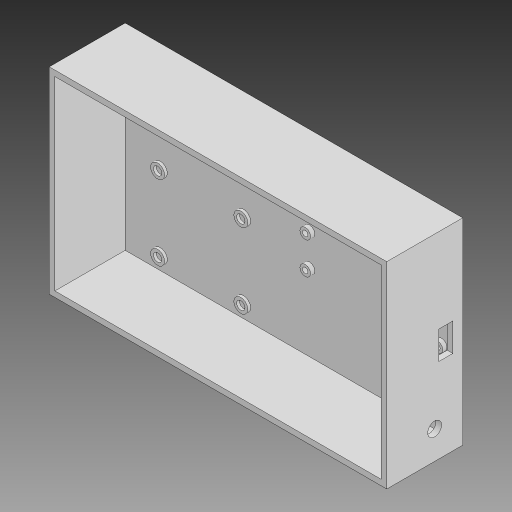
# Autodesk Inventor part: box
Saved by Autodesk Inventor 2023 (Build 270158000, 158)
## iProperties
Created: 2024-01-29
Part Number: box
Material: Všeobecné
Document SubType Name: Modeling
Designer: matej
Mass: 35.3602 g
Surface Area: 363.22 cm^2
Volume: 35.3602 cm^3
Density: 1 g/cm^3
Appearance: Výchozí
Author: matej
Autodesk Inventor part; units mm, degrees
ref_plane "YZ Plane" through (0, 0, 0) normal (1, 0, 0) x (0, 1, 0)
ref_plane "XZ Plane" through (0, 0, 0) normal (0, 1, 0) x (-1, 0, 0)
ref_plane "XY Plane" through (0, 0, 0) normal (0, 0, 1) x (1, 0, 0)
sketch "Náčrt1" plane through (0, 0, 0) normal (0, 0, 1) x (1, 0, 0)
  line L0 (-60, -35) -> (60, -35)
  line L1 (60, -35) -> (60, 35)
  line L2 (60, 35) -> (-60, 35)
  line L3 (-60, 35) -> (-60, -35)
  line L4 (-60, -35) -> (60, 35) construction
  line L5 (60, -35) -> (-60, 35) construction
  point P0 (0, 0)
  dimension "d0" = 120
  dimension "d1" = 70
  constraints: 12 end point, 2 midpoint, 2 parallel, 1 horizontal, 1 perpendicular
  measures "d0" distance of L2.end L1.end
  measures "d1" distance of L1.end L0.end
extrude "Vysunutí1" add sketch "Náčrt1" along normal blind 2
sketch "Náčrt2" plane through (0, 0, 2) normal (0, 0, 1) x (1, 0, 0)
  line L0 (60, -35) -> (60, 35) projected
  line L1 (-60, -35) -> (60, -35)
  line L2 (60, -35) -> (60, 35)
  line L3 (60, 35) -> (-60, 35)
  line L4 (-60, 35) -> (-60, -35)
  line L5 (-60, -35) -> (60, 35) construction
  line L6 (60, -35) -> (-60, 35) construction
  line L7 (-58, -33) -> (58, -33)
  line L8 (58, -33) -> (58, 33)
  line L9 (58, 33) -> (-58, 33)
  line L10 (-58, 33) -> (-58, -33)
  line L11 (-58, -33) -> (58, 33) construction
  line L12 (58, -33) -> (-58, 33) construction
  point P0 (0, 0)
  point P1 (60, -35)
  dimension "d4" = 116
  dimension "d5" = 66
  constraints: 24 end point, 4 midpoint, 4 parallel, 2 horizontal, 2 perpendicular
  measures "d4" distance of L9.end L8.end
  measures "d5" distance of L8.end L7.end
extrude "Vysunutí2" add sketch "Náčrt2" along normal blind 25
sketch "Náčrt3" plane through (60, -35, 0) normal (1, 0, 0) x (0, 0, -1)
  line L0 (-8.5, 30) -> (-3.5, 30)
  line L1 (-3.5, 30) -> (-3.5, 40)
  line L2 (-3.5, 40) -> (-8.5, 40)
  line L3 (-8.5, 40) -> (-8.5, 30)
  line L4 (-8.5, 30) -> (-3.5, 40) construction
  line L5 (-3.5, 30) -> (-8.5, 40) construction
  line L6 (0, 0) -> (0, 70) projected
  point P0 (0, 35)
  point P1 (-6, 35)
  point P2 (0, 35)
  dimension "d8" = 3.5
  dimension "d9" = 5
  dimension "d10" = 10
  constraints: 12 end point, 3 midpoint, 2 parallel, 1 horizontal, 1 horizontal alignment, 1 perpendicular
  measures "d8" distance between parallel lines of L1 L6
  measures "d9" distance of L0.start L0.end
  measures "d10" distance of L2.end L0.start
extrude "micro usb hole" cut sketch "Náčrt3" against normal blind 5
sketch "Náčrt4" plane through (0, 0, 2) normal (0, 0, 1) x (1, 0, 0)
  circle A0 centre (54.5, 5.7) radius 1.9
  circle A1 centre (54.5, -5.7) radius 1.9
  circle A2 centre (7.5, 5.7) radius 1.9
  circle A3 centre (7.5, -5.7) radius 1.9
  line L0 (5.5, 10.5) -> (56.5, 10.5)
  line L1 (56.5, 10.5) -> (56.5, -10.5)
  line L2 (56.5, -10.5) -> (5.5, -10.5)
  line L3 (5.5, -10.5) -> (5.5, 10.5)
  line L4 (60, -35) -> (60, 35) projected
  line L5 (58, 33) -> (58, -33) projected
  circle A4 centre (54.5, 5.7) radius 1
  circle A5 centre (7.5, 5.7) radius 1
  circle A6 centre (7.5, -5.7) radius 1
  circle A7 centre (54.5, -5.7) radius 1
  point P0 (0, 0)
  point P1 (56.5, 0)
  point P2 (60, 0)
  dimension "d13" = 3.8
  dimension "d14" = 3.8
  dimension "d15" = 11.4
  dimension "d16" = 3.8
  dimension "d18" = 3.8
  dimension "d19" = 51
  dimension "d20" = 2
  dimension "d21" = 2
  dimension "d22" = 21
  dimension "d23" = 4.8
  dimension "d24" = 1.5
  dimension "d25" = 2
  dimension "d26" = 2
  dimension "d27" = 2
  dimension "d28" = 2
  constraints: 8 centre point, 8 end point, 4 coincident, 3 horizontal alignment, 2 midpoint, 2 parallel, 2 vertical alignment, 1 horizontal, 1 perpendicular
  measures "d13" diameter of A0
  measures "d14" diameter of A1
  measures "d15" distance of A1.centre A0.centre
  measures "d16" diameter of A2
  measures "d18" diameter of A3
  measures "d19" distance of L0.start L0.end
  measures "d20" distance from line of L1 A0.centre
  measures "d21" distance from line of L3 A2.centre
  measures "d22" distance of L2.end L0.start
  measures "d23" distance from line of L0 A0.centre
  measures "d24" distance between parallel lines of L5 L1
  measures "d25" diameter of A4
  measures "d26" diameter of A5
  measures "d27" diameter of A6
  measures "d28" diameter of A7
extrude "rpi holder" add sketch "Náčrt4" along normal blind 1.5 contours A0 | A1 | A2 | A3
sketch "Náčrt6" plane through (60, -35, 0) normal (1, 0, 0) x (0, 0, -1)
  circle A0 centre (-10, 10) radius 2.5
  line L0 (0, 70) -> (-27, 70) projected
  line L1 (0, 0) -> (0, 70) projected
  line L2 (0, 0) -> (-27, 0) projected
  point P0 (0, 35)
  dimension "d36" = 5
  dimension "d38" = 10
  dimension "d59" = 10
  constraints: 1 centre point
  measures "d36" diameter of A0
  measures "d38" distance from line of L1 A0.centre
  measures "d59" distance from line of L2 A0.centre
extrude "rgb led hole" cut sketch "Náčrt6" against normal blind 10
sketch "Náčrt7" plane through (0, 0, 2) normal (0, 0, 1) x (1, 0, 0)
  line L0 (-48, 0.8) -> (-13.4, 0.8)
  line L1 (-13.4, 0.8) -> (-13.4, -31)
  line L2 (-13.4, -31) -> (-48, -31)
  line L3 (-48, -31) -> (-48, 0.8)
  circle A0 centre (-15.9, -1.8) radius 1.5
  circle A1 centre (-45.5, -1.8) radius 2.5
  circle A2 centre (-45.5, -28.4) radius 1.5
  circle A3 centre (-15.9, -28.4) radius 1.5
  circle A4 centre (-45.5, -1.8) radius 1.5
  circle A5 centre (-15.9, -1.8) radius 2.5
  circle A6 centre (-15.9, -28.4) radius 2.5
  circle A7 centre (-45.5, -28.4) radius 2.5
  line L4 (-58, -33) -> (-58, 33) projected
  line L5 (58, -33) -> (-58, -33) projected
  point P0 (0, 0)
  point P1 (-48, -1.8)
  point P2 (-48, -28.4)
  point P3 (-13.4, -28.4)
  point P4 (-13.4, -1.8)
  dimension "d41" = 34.6
  dimension "d42" = 31.8
  dimension "d43" = 3
  dimension "d44" = 5
  dimension "d45" = 29.6
  dimension "d46" = 2.5
  dimension "d47" = 2.6
  dimension "d48" = 3
  dimension "d49" = 3
  dimension "d50" = 26.6
  dimension "d51" = 3
  dimension "d52" = 5
  dimension "d53" = 5
  dimension "d54" = 5
  dimension "d55" = 10
  dimension "d56" = 2
  constraints: 8 centre point, 8 end point, 4 coincident, 2 horizontal alignment, 2 parallel, 2 vertical alignment, 1 horizontal, 1 perpendicular
  measures "d41" distance of L1.end L2.end
  measures "d42" distance of L0.end L1.end
  measures "d43" diameter of A0
  measures "d44" diameter of A1
  measures "d45" distance of A1.centre A0.centre
  measures "d46" distance from line of L1 A0.centre
  measures "d47" distance from line of L0 A0.centre
  measures "d48" diameter of A2
  measures "d49" diameter of A3
  measures "d50" distance of A0.centre A3.centre
  measures "d51" diameter of A4
  measures "d52" diameter of A5
  measures "d53" diameter of A6
  measures "d54" diameter of A7
  measures "d55" distance between parallel lines of L4 L3
  measures "d56" distance between parallel lines of L5 L2
extrude "ULN2003 holder" add sketch "Náčrt7" along normal blind 1 contours A1 | A7 | A6 | A5
equation "\"d14\" = d13"
equation "\"d16\" = d13"
equation "\"d18\" = d13"
equation "\"d26\" = d25"
equation "\"d27\" = d25"
equation "\"d28\" = d25"
equation "\"d43\" = d49"
equation "\"d44\" = d53"
equation "\"d48\" = d49"
equation "\"d51\" = d49"
equation "\"d52\" = d53"
equation "\"d54\" = d53"
